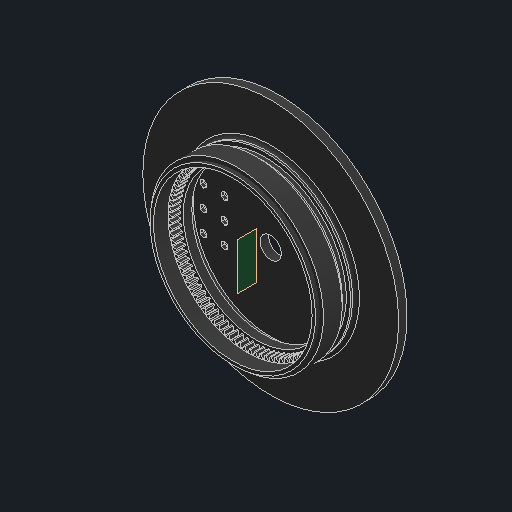
# Autodesk Inventor part: 스퍼 기어1
Saved by Autodesk Inventor 2026.1 (Build 301233020, 233B)
## iProperties
CustomPartVersion: 1
Created: 2025-11-12
Part Number: 스퍼 기어1
Material: 고무, 검은색
Document SubType Name: Modeling
Designer: jaewook
Categories: <?xml version="1.0" encoding="UTF-16"?> <MemberInstance><Categories><FamilyTemplate><FamilyTemplateParameter ValueType="xs:double" Id="1" ObjectReferenceKey="da_z" ObjectType="kUserParameterObject"/><FamilyTemplateParameter ValueType="xs:double" Id="2" ObjectReferenceKey="da_b" ObjectType="kUserParameterObject"/><FamilyTemplateParameter ValueType="xs:double" Id="3" ObjectReferenceKey="da_beta" ObjectType="kUserParameterObject"/><FamilyTemplateParameter ValueType="xs:double" Id="4" ObjectReferenceKey="da_da" ObjectType="kUserParameterObject"/><FamilyTemplateParameter ValueType="xs:double" Id="5" ObjectReferenceKey="da_aw" ObjectType="kUserParameterObject"/><FamilyTemplateParameter ValueType="xs:string" Id="6" ObjectReferenceKey="EAIAABAAAACIAQAAAAAAAIAAAAAAAAAA" ObjectType="83910656" SubObjectId="SurfaceGeometry"/></FamilyTemplate><ParamToTemplateMap><ParamToTemplate CategoryParameter="//CategoryParameter[@InternalName='046C89C9-8512-4d59-83FE-43B91F4F132A']" TemplateParameter="1"/><ParamToTemplate CategoryParameter="//CategoryParameter[@InternalName='2552DF32-E462-4b46-AEBF-C6C7768E72AC']" TemplateParameter="2"/><ParamToTemplate CategoryParameter="//CategoryParameter[@InternalName='C9EE641D-15FC-4fae-A226-E94C4372FDD7']" TemplateParameter="3"/><ParamToTemplate><ParamToTemplate CategoryParameter="//CategoryParameter[@InternalName='00B6519A-459B-49c7-AD84-2E56D39A5744']" ConstantValue="0.000000"/></ParamToTemplate><ParamToTemplate><ParamToTemplate CategoryParameter="//CategoryParameter[@InternalName='04B31F0E-C7A6-4894-AA32-9629BEFACF47']" ConstantValue="0.950000"/></ParamToTemplate><ParamToTemplate><ParamToTemplate CategoryParameter="//CategoryParameter[@InternalName='43CBEC2E-7847-49e7-A936-2F7889FCB2D9']" ConstantValue="0.250000"/></ParamToTemplate><ParamToTemplate><ParamToTemplate CategoryParameter="//CategoryParameter[@InternalName='B1EFC894-105D-4ebd-86BF-FA20ED196853']" ConstantValue="0.379900"/></ParamToTemplate><ParamToTemplate><ParamToTemplate CategoryParameter="//CategoryParameter[@InternalName='51175063-3D10-4879-93E8-6246FE8B403D']" ConstantValue="2060000000.000000"/></ParamToTemplate><ParamToTemplate><ParamToTemplate CategoryParameter="//CategoryParameter[@InternalName='A3A52E27-4454-46a9-B0BD-C932399B70AF']" ConstantValue="0.300000"/></ParamToTemplate><ParamToTemplate><ParamToTemplate CategoryParameter="//CategoryParameter[@InternalName='91B76062-C214-41d9-B1B9-14D2AB99603D']" ConstantValue="0.200000"/></ParamToTemplate><ParamToTemplate><ParamToTemplate CategoryParameter="//CategoryParameter[@InternalName='374E806E-8B8A-4dda-A9AA-1039D6500AD2']" ConstantValue="5.000000"/></ParamToTemplate><ParamToTemplate><ParamToTemplate CategoryParameter="//CategoryParameter[@InternalName='2D373A89-B862-43d6-8D0B-0CBF12AB9F6C']" ConstantValue="0.349066"/></ParamToTemplate><ParamToTemplate CategoryParameter="//CategoryParameter[@InternalName='37777632-D6A2-4fac-9D53-DB8ACD95C989']" TemplateParameter="4"/><ParamToTemplate CategoryParameter="//CategoryParameter[@InternalName='FD1017F1-B727-4f7e-9707-0F86F1FF9423']" TemplateParameter="5"/><ParamToTemplate><ParamToTemplate CategoryParameter="//CategoryParameter[@InternalName='9E1B4470-B2D3-4ff1-B813-535BB4CDF51A']" ConstantValue="3520000.000000"/></ParamToTemplate><ParamToTemplate><ParamToTemplate CategoryParameter="//CategoryParameter[@InternalName='F8452263-BFF6-458c-9FB1-07C4B99E95CD']" ConstantValue="11400000.000000"/></ParamToTemplate><ParamToTemplate><ParamToTemplate CategoryParameter="//CategoryParameter[@InternalName='3E3BB259-FD49-497f-8171-6EBC954A3479']" ConstantValue="2.000000"/></ParamToTemplate><ParamToTemplate CategoryParameter="//CategoryParameter[@InternalName='27C3BAF2-7550-4e4b-AE2C-0DB134B7D9B7']" TemplateParameter="6"/></ParamToTemplateMap><Category DisplayName="Gear" InternalName="DC85795E-93AB-48d5-8EEE-5A27447B64BD" Mnemonic="Gear"><CategoryParameter DisplayName="z" InternalName="046C89C9-8512-4d59-83FE-43B91F4F132A" Mnemonic="z"/><CategoryParameter DisplayName="b" InternalName="2552DF32-E462-4b46-AEBF-C6C7768E72AC" Mnemonic="b"/><CategoryParameter DisplayName="||b|" InternalName="C9EE641D-15FC-4fae-A226-E94C4372FDD7" Mnemonic="beta"/><CategoryParameter DisplayName="x" InternalName="00B6519A-459B-49c7-AD84-2E56D39A5744" Mnemonic="x"/><CategoryParameter DisplayName="a*" InternalName="04B31F0E-C7A6-4894-AA32-9629BEFACF47" Mnemonic="a"/><CategoryParameter DisplayName="c*" InternalName="43CBEC2E-7847-49e7-A936-2F7889FCB2D9" Mnemonic="c"/><CategoryParameter DisplayName="r|.f|*" InternalName="B1EFC894-105D-4ebd-86BF-FA20ED196853" Mnemonic="rf"/><CategoryParameter DisplayName="E" InternalName="51175063-3D10-4879-93E8-6246FE8B403D" Mnemonic="E"/><CategoryParameter DisplayName="||m|" InternalName="A3A52E27-4454-46a9-B0BD-C932399B70AF" Mnemonic="mi"/><Category DisplayName="SpurGear" InternalName="26C5A22E-A91E-4dfd-A3B3-23CCAFAE1764" Mnemonic="SpurGear"><CategoryParameter DisplayName="m" InternalName="91B76062-C214-41d9-B1B9-14D2AB99603D" Mnemonic="m"/><CategoryParameter DisplayName="P" InternalName="374E806E-8B8A-4dda-A9AA-1039D6500AD2" Mnemonic="PP"/><CategoryParameter DisplayName="||a|" InternalName="2D373A89-B862-43d6-8D0B-0CBF12AB9F6C" Mnemonic="alpha"/><CategoryParameter DisplayName="d|.a|" InternalName="37777632-D6A2-4fac-9D53-DB8ACD95C989" Mnemonic="da"/><CategoryParameter DisplayName="a|.w|" InternalName="FD1017F1-B727-4f7e-9707-0F86F1FF9423" Mnemonic="aw"/><CategoryParameter DisplayName="||s||.Flim|" InternalName="9E1B4470-B2D3-4ff1-B813-535BB4CDF51A" Mnemonic="sFlim"/><CategoryParameter DisplayName="||s||.Hlim|" InternalName="F8452263-BFF6-458c-9FB1-07C4B99E95CD" Mnemonic="sHlim"/><CategoryParameter DisplayName="유형" InternalName="3E3BB259-FD49-497f-8171-6EBC954A3479" Mnemonic="type"/><Category DisplayName="InternalSpurGear" InternalName="7CF704F6-14A9-42f8-93CE-E71DF57C2B55" Mnemonic="InternalSpurGear"><CategoryParameter DisplayName="PitchDiameter" InternalName="27C3BAF2-7550-4e4b-AE2C-0DB134B7D9B7" Mnemonic="IDS_PITCHDIAM"/></Category></Category></Category></Categories></MemberInstance>
Density: 0.93 g/cm^3
Appearance: 고무 - 검은색
d16: 70.000 mm
d17: 0.000 mm
d45: 0.000 mm
d47: 70.000 mm
d50: 0.000 mm
d51: 0.000 mm
d52: 70.000 mm
Author: jaewook
Autodesk Inventor part; units mm, degrees
sketch "Sketch1" plane through (0, 0, 0) normal (0, 0, 1) x (1, 0, 0)
  circle A0 centre (0, 0) radius 97.02
  dimension "d0" = 194.04
  constraints: 1 centre point
  measures "d0" diameter of A0
extrude "Extrusion1" add sketch "Sketch1" along normal blind 10
ref_plane "Work Plane2" through (0, 0, 5) normal (0, 0, 1) x (1, 0, 0)
sketch "Sketch2" plane through (0, 0, 0) normal (0, 0, -1) x (-1, 0, 0)
  circle A0 centre (0, 0) radius 97.02 projected
  circle A1 centre (0, 0) radius 90
  dimension "d3" = 180
  constraints: 1 centre point, 1 coincident
  measures "d3" diameter of A1
surface extrude "피치 지름" sketch "Sketch2" against normal through all shown no curves A1
ref_plane "Work Plane8" through (0, 0, 0) normal (0.9993908, 0.0348995, 0) x (0, 0, 1)
ref_plane "Work Plane9" through (0, 0, 0) normal (1, 0, 0) x (0, 1, 0)
spur gear teeth "스퍼 기어" teeth 90 pitch diameter 180 tip diameter 176.2 root diameter 184.8 face width 10 start plane through (0, 0, 0) normal (0, 0, -1) x (-1, 0, 0)
sketch "스케치14" plane through (0, 0, 10) normal (0, 0, 1) x (1, 0, 0)
  circle A0 centre (0, 0) radius 97.02 projected
  circle A1 centre (0, 0) radius 93.02
  dimension "d81" = 4
  constraints: 1 centre point, 1 coincident
  measures "d81" radial gap between concentric circles of A1 A0
extrude "돌출9" add sketch "스케치14" along normal blind 17
sketch "스케치15" plane through (0, 0, 0) normal (0, 0, -1) x (-1, 0, 0)
  circle A0 centre (0, 0) radius 97.02 projected
  circle A1 centre (0, 0) radius 92.4
  circle A2 centre (0, 0) radius 95.02
  circle A3 centre (0, 0) radius 85
  dimension "d84" = 184.8
  dimension "d85" = 190.04
  dimension "d86" = 170
  constraints: 3 centre point, 3 coincident
  measures "d84" diameter of A1
  measures "d85" diameter of A2
  measures "d86" diameter of A3
extrude "돌출10" add sketch "스케치15" along normal blind 10 contours A1 | A2
sketch "스케치16" plane through (0, 0, -10) normal (0, 0, -1) x (-1, 0, 0)
  circle A0 centre (0, 0) radius 95.02 projected
  circle A1 centre (0, 0) radius 85 projected
  circle A2 centre (0, 0) radius 90.78
  dimension "d89" = 4.24
  constraints: 1 centre point, 1 coincident
  measures "d89" radial gap between concentric circles of A2 A0
extrude "돌출11" add sketch "스케치16" along normal blind 1 contours A0
sketch "스케치17" plane through (0, 0, -11) normal (0, 0, -1) x (-1, 0, 0)
  circle A0 centre (0, 0) radius 90.78 projected
  circle A1 centre (0, 0) radius 85 projected
  circle A2 centre (0, 0) radius 100.02
  circle A3 centre (0, 0) radius 95.02 projected
  dimension "d150" = 5
  constraints: 1 centre point, 1 coincident
  measures "d150" radial gap between concentric circles of A2 A3
extrude "돌출12" add sketch "스케치17" along normal blind 6.5 contours A2 | A3
sketch "스케치18" plane through (0, 0, -17.5) normal (0, 0, -1) x (-1, 0, 0)
  circle A0 centre (0, 0) radius 90.78 projected
  circle A1 centre (0, 0) radius 150
  circle A2 centre (0, 0) radius 12.5
  dimension "d94" = 300
  dimension "d95" = 25
  constraints: 2 centre point, 2 coincident
  measures "d94" diameter of A1
  measures "d95" diameter of A2
extrude "돌출13" add sketch "스케치18" along normal blind 10 contours A0 | A1
fillet "모깎기2" radius 4 1 edges at (100.02, 0, -17.5)
sketch "스케치4" plane through (0, 0, 0) normal (0, 0, -1) x (-1, 0, 0)
  arc A0 (-13.6576, -91.3851) -> (-12.0606, -91.6095) centre (0, 0) ccw projected
  arc A1 (-19.999, -90.2098) -> (-18.4216, -90.545) centre (0, 0) ccw projected
  arc A2 (-26.243, -88.5949) -> (-24.6928, -89.0395) centre (0, 0) ccw projected
  arc A3 (-32.3592, -86.5485) -> (-30.8438, -87.1001) centre (0, 0) ccw projected
  arc A4 (-38.3177, -84.0804) -> (-36.8444, -84.7364) centre (0, 0) ccw projected
  arc A5 (-44.0895, -81.2027) -> (-42.6656, -81.9598) centre (0, 0) ccw projected
  arc A6 (-49.6465, -77.9294) -> (-48.2789, -78.784) centre (0, 0) ccw projected
  arc A7 (-54.9616, -74.2764) -> (-53.657, -75.2243) centre (0, 0) ccw projected
  arc A8 (-60.009, -70.2615) -> (-58.7736, -71.2981) centre (0, 0) ccw projected
  arc A9 (-64.764, -65.9043) -> (-63.604, -67.0246) centre (0, 0) ccw projected
  arc A10 (-69.2035, -61.2261) -> (-68.1244, -62.4245) centre (0, 0) ccw projected
  arc A11 (-73.3058, -56.2496) -> (-72.313, -57.5204) centre (0, 0) ccw projected
  arc A12 (-77.051, -50.999) -> (-76.1493, -52.3359) centre (0, 0) ccw projected
  arc A13 (-80.4209, -45.4999) -> (-79.6145, -46.8965) centre (0, 0) ccw projected
  arc A14 (-83.3989, -39.7792) -> (-82.6919, -41.2287) centre (0, 0) ccw projected
  arc A15 (-85.9706, -33.8647) -> (-85.3665, -35.3599) centre (0, 0) ccw projected
  arc A16 (-88.1234, -27.7852) -> (-87.6251, -29.319) centre (0, 0) ccw projected
  arc A17 (-89.847, -21.5704) -> (-89.4568, -23.1351) centre (0, 0) ccw projected
  arc A18 (-91.1328, -15.2504) -> (-90.8528, -16.8386) centre (0, 0) ccw projected
  arc A19 (-91.9746, -8.8561) -> (-91.806, -10.46) centre (0, 0) ccw projected
  arc A20 (-92.3683, -2.4188) -> (-92.3121, -4.0304) centre (0, 0) ccw projected
  arc A21 (-92.3121, 4.0304) -> (-92.3683, 2.4188) centre (0, 0) ccw projected
  arc A22 (-91.806, 10.46) -> (-91.9746, 8.8561) centre (0, 0) ccw projected
  arc A23 (-90.8528, 16.8386) -> (-91.1328, 15.2504) centre (0, 0) ccw projected
  arc A24 (-89.4568, 23.1351) -> (-89.847, 21.5704) centre (0, 0) ccw projected
  arc A25 (-87.6251, 29.319) -> (-88.1234, 27.7852) centre (0, 0) ccw projected
  arc A26 (-85.3665, 35.3599) -> (-85.9706, 33.8647) centre (0, 0) ccw projected
  arc A27 (-82.6919, 41.2287) -> (-83.3989, 39.7792) centre (0, 0) ccw projected
  arc A28 (-79.6145, 46.8965) -> (-80.4209, 45.4999) centre (0, 0) ccw projected
  arc A29 (-76.1493, 52.3359) -> (-77.051, 50.999) centre (0, 0) ccw projected
  arc A30 (-72.313, 57.5204) -> (-73.3058, 56.2496) centre (0, 0) ccw projected
  arc A31 (-68.1244, 62.4245) -> (-69.2035, 61.2261) centre (0, 0) ccw projected
  arc A32 (-63.604, 67.0246) -> (-64.764, 65.9043) centre (0, 0) ccw projected
  arc A33 (-58.7736, 71.2981) -> (-60.009, 70.2615) centre (0, 0) ccw projected
  arc A34 (-53.657, 75.2243) -> (-54.9616, 74.2764) centre (0, 0) ccw projected
  arc A35 (-48.2789, 78.784) -> (-49.6465, 77.9294) centre (0, 0) ccw projected
  arc A36 (-42.6656, 81.9598) -> (-44.0895, 81.2027) centre (0, 0) ccw projected
  arc A37 (-36.8444, 84.7364) -> (-38.3177, 84.0804) centre (0, 0) ccw projected
  arc A38 (-30.8438, 87.1001) -> (-32.3592, 86.5485) centre (0, 0) ccw projected
  arc A39 (-24.6928, 89.0395) -> (-26.243, 88.5949) centre (0, 0) ccw projected
  arc A40 (-18.4216, 90.545) -> (-19.999, 90.2098) centre (0, 0) ccw projected
  arc A41 (-12.0606, 91.6095) -> (-13.6576, 91.3851) centre (0, 0) ccw projected
  arc A42 (-5.6409, 92.2277) -> (-7.2496, 92.1152) centre (0, 0) ccw projected
  arc A43 (0.8063, 92.3965) -> (-0.8063, 92.3965) centre (0, 0) ccw projected
  arc A44 (7.2496, 92.1152) -> (5.6409, 92.2277) centre (0, 0) ccw projected
  arc A45 (13.6576, 91.3851) -> (12.0606, 91.6095) centre (0, 0) ccw projected
  arc A46 (19.999, 90.2098) -> (18.4216, 90.545) centre (0, 0) ccw projected
  arc A47 (26.243, 88.5949) -> (24.6928, 89.0395) centre (0, 0) ccw projected
  arc A48 (32.3592, 86.5485) -> (30.8438, 87.1001) centre (0, 0) ccw projected
  arc A49 (38.3177, 84.0804) -> (36.8444, 84.7364) centre (0, 0) ccw projected
  arc A50 (44.0895, 81.2027) -> (42.6656, 81.9598) centre (0, 0) ccw projected
  arc A51 (49.6465, 77.9294) -> (48.2789, 78.784) centre (0, 0) ccw projected
  arc A52 (54.9616, 74.2764) -> (53.657, 75.2243) centre (0, 0) ccw projected
  arc A53 (60.009, 70.2615) -> (58.7736, 71.2981) centre (0, 0) ccw projected
  arc A54 (64.764, 65.9043) -> (63.604, 67.0246) centre (0, 0) ccw projected
  arc A55 (69.2035, 61.2261) -> (68.1244, 62.4245) centre (0, 0) ccw projected
  arc A56 (73.3058, 56.2496) -> (72.313, 57.5204) centre (0, 0) ccw projected
  arc A57 (77.051, 50.999) -> (76.1493, 52.3359) centre (0, 0) ccw projected
  arc A58 (80.4209, 45.4999) -> (79.6145, 46.8965) centre (0, 0) ccw projected
  arc A59 (83.3989, 39.7792) -> (82.6919, 41.2287) centre (0, 0) ccw projected
  arc A60 (85.9706, 33.8647) -> (85.3665, 35.3599) centre (0, 0) ccw projected
  arc A61 (88.1234, 27.7852) -> (87.6251, 29.319) centre (0, 0) ccw projected
  arc A62 (89.847, 21.5704) -> (89.4568, 23.1351) centre (0, 0) ccw projected
  arc A63 (91.1328, 15.2504) -> (90.8528, 16.8386) centre (0, 0) ccw projected
  arc A64 (91.9746, 8.8561) -> (91.806, 10.46) centre (0, 0) ccw projected
  arc A65 (92.3683, 2.4188) -> (92.3121, 4.0304) centre (0, 0) ccw projected
  arc A66 (92.3121, -4.0304) -> (92.3683, -2.4188) centre (0, 0) ccw projected
  arc A67 (91.806, -10.46) -> (91.9746, -8.8561) centre (0, 0) ccw projected
  arc A68 (90.8528, -16.8386) -> (91.1328, -15.2504) centre (0, 0) ccw projected
  arc A69 (89.4568, -23.1351) -> (89.847, -21.5704) centre (0, 0) ccw projected
  arc A70 (87.6251, -29.319) -> (88.1234, -27.7852) centre (0, 0) ccw projected
  arc A71 (85.3665, -35.3599) -> (85.9706, -33.8647) centre (0, 0) ccw projected
  arc A72 (82.6919, -41.2287) -> (83.3989, -39.7792) centre (0, 0) ccw projected
  arc A73 (79.6145, -46.8965) -> (80.4209, -45.4999) centre (0, 0) ccw projected
  arc A74 (76.1493, -52.3359) -> (77.051, -50.999) centre (0, 0) ccw projected
  arc A75 (72.313, -57.5204) -> (73.3058, -56.2496) centre (0, 0) ccw projected
  arc A76 (68.1244, -62.4245) -> (69.2035, -61.2261) centre (0, 0) ccw projected
  arc A77 (63.604, -67.0246) -> (64.764, -65.9043) centre (0, 0) ccw projected
  arc A78 (58.7736, -71.2981) -> (60.009, -70.2615) centre (0, 0) ccw projected
  arc A79 (53.657, -75.2243) -> (54.9616, -74.2764) centre (0, 0) ccw projected
  arc A80 (48.2789, -78.784) -> (49.6465, -77.9294) centre (0, 0) ccw projected
  arc A81 (42.6656, -81.9598) -> (44.0895, -81.2027) centre (0, 0) ccw projected
  arc A82 (36.8444, -84.7364) -> (38.3177, -84.0804) centre (0, 0) ccw projected
  arc A83 (30.8438, -87.1001) -> (32.3592, -86.5485) centre (0, 0) ccw projected
  arc A84 (24.6928, -89.0395) -> (26.243, -88.5949) centre (0, 0) ccw projected
  arc A85 (18.4216, -90.545) -> (19.999, -90.2098) centre (0, 0) ccw projected
  arc A86 (12.0606, -91.6095) -> (13.6576, -91.3851) centre (0, 0) ccw projected
  arc A87 (5.6409, -92.2277) -> (7.2496, -92.1152) centre (0, 0) ccw projected
  arc A88 (-0.8063, -92.3965) -> (0.8063, -92.3965) centre (0, 0) ccw projected
  arc A89 (-7.2496, -92.1152) -> (-5.6409, -92.2277) centre (0, 0) ccw projected
  circle A90 centre (0, 0) radius 97.02 projected
  circle A91 centre (0, 0) radius 92.4
  point P0 (-92.3683, 2.4188)
  point P1 (-92.3121, 4.0304)
  point P2 (-91.9746, 8.8561)
  point P3 (-91.1328, 15.2504)
  point P4 (-89.847, 21.5704)
  point P5 (-88.1234, 27.7852)
  point P6 (-83.3989, 39.7792)
  point P7 (-80.4209, 45.4999)
  point P8 (-79.6145, 46.8965)
  point P9 (-76.1493, 52.3359)
  point P10 (-72.313, 57.5204)
  point P11 (-60.009, 70.2615)
  point P12 (-58.7736, 71.2981)
  point P13 (-54.9616, 74.2764)
  point P14 (-53.657, 75.2243)
  point P15 (-44.0895, 81.2027)
  point P16 (-38.3177, 84.0804)
  point P17 (-32.3592, 86.5485)
  point P18 (-26.243, 88.5949)
  point P19 (-24.6928, 89.0395)
  point P20 (-19.999, 90.2098)
  point P21 (-18.4216, 90.545)
  point P22 (-13.6576, 91.3851)
  point P23 (-12.0606, 91.6095)
  point P24 (-7.2496, 92.1152)
  point P25 (-0.8063, 92.3965)
  point P26 (0.8063, 92.3965)
  point P27 (5.6409, 92.2277)
  point P28 (7.2496, 92.1152)
  point P29 (12.0606, 91.6095)
  point P30 (18.4216, 90.545)
  point P31 (24.6928, 89.0395)
  point P32 (30.8438, 87.1001)
  point P33 (36.8444, 84.7364)
  point P34 (38.3177, 84.0804)
  point P35 (42.6656, 81.9598)
  point P36 (48.2789, 78.784)
  point P37 (49.6465, 77.9294)
  point P38 (54.9616, 74.2764)
  point P39 (58.7736, 71.2981)
  point P40 (63.604, 67.0246)
  point P41 (68.1244, 62.4245)
  point P42 (72.313, 57.5204)
  point P43 (73.3058, 56.2496)
  point P44 (79.6145, 46.8965)
  point P45 (80.4209, 45.4999)
  point P46 (85.3665, 35.3599)
  point P47 (87.6251, 29.319)
  point P48 (89.4568, 23.1351)
  point P49 (89.847, 21.5704)
  point P50 (90.8528, 16.8386)
  point P51 (91.1328, 15.2504)
  point P52 (91.806, 10.46)
  point P53 (91.9746, 8.8561)
  point P54 (92.3683, -2.4188)
  point P55 (92.3121, -4.0304)
  point P56 (91.9746, -8.8561)
  point P57 (91.1328, -15.2504)
  point P58 (89.847, -21.5704)
  point P59 (88.1234, -27.7852)
  point P60 (85.9706, -33.8647)
  point P61 (72.313, -57.5204)
  point P62 (60.009, -70.2615)
  point P63 (58.7736, -71.2981)
  point P64 (54.9616, -74.2764)
  point P65 (53.657, -75.2243)
  point P66 (49.6465, -77.9294)
  point P67 (44.0895, -81.2027)
  point P68 (38.3177, -84.0804)
  point P69 (32.3592, -86.5485)
  point P70 (26.243, -88.5949)
  point P71 (19.999, -90.2098)
  point P72 (18.4216, -90.545)
  point P73 (13.6576, -91.3851)
  point P74 (12.0606, -91.6095)
  point P75 (7.2496, -92.1152)
  point P76 (0.8063, -92.3965)
  point P77 (-0.8063, -92.3965)
  point P78 (-7.2496, -92.1152)
  point P79 (-12.0606, -91.6095)
  point P80 (-18.4216, -90.545)
  point P81 (-24.6928, -89.0395)
  point P82 (-26.243, -88.5949)
  point P83 (-30.8438, -87.1001)
  point P84 (-32.3592, -86.5485)
  point P85 (-36.8444, -84.7364)
  point P86 (-38.3177, -84.0804)
  point P87 (-48.2789, -78.784)
  point P88 (-53.657, -75.2243)
  point P89 (-58.7736, -71.2981)
  point P90 (-63.604, -67.0246)
  point P91 (-64.764, -65.9043)
  point P92 (-69.2035, -61.2261)
  point P93 (-72.313, -57.5204)
  point P94 (-73.3058, -56.2496)
  point P95 (-76.1493, -52.3359)
  point P96 (-77.051, -50.999)
  point P97 (-82.6919, -41.2287)
  point P98 (-83.3989, -39.7792)
  point P99 (-85.3665, -35.3599)
  point P100 (-87.6251, -29.319)
  point P101 (-90.8528, -16.8386)
  point P102 (-91.806, -10.46)
  point P103 (-92.3121, -4.0304)
  constraints: 1 coincident, 1 other
sketch "스케치6" plane through (0, 0, -10) normal (0, 0, -1) x (-1, 0, 0)
  arc A0 (51.6266, -76.6319) -> (92.1785, -6.394) centre (0, 0) ccw projected
  circle A1 centre (0, 0) radius 101.64 projected
  arc A2 (92.1785, 6.394) -> (51.6266, 76.6319) centre (0, 0) ccw projected
  circle A3 centre (0, 0) radius 97.02
  dimension "d69" = 4.62
  constraints: 1 centre point, 1 coincident
  measures "d69" radial gap between concentric circles of A0 A3
sketch "스케치7" plane through (0, 0, -10) normal (0, 0, -1) x (-1, 0, 0)
  circle A0 centre (0, 0) radius 97.02 projected
  arc A1 (51.6266, -76.6319) -> (92.1785, -6.394) centre (0, 0) ccw projected
  arc A2 (-40.5519, -83.0259) -> (40.5519, -83.0259) centre (0, 0) ccw projected
  arc A3 (-92.1785, -6.394) -> (-51.6266, -76.6319) centre (0, 0) ccw projected
  arc A4 (-51.6266, 76.6319) -> (-92.1785, 6.394) centre (0, 0) ccw projected
  arc A5 (40.5519, 83.0259) -> (-40.5519, 83.0259) centre (0, 0) ccw projected
  arc A6 (92.1785, 6.394) -> (51.6266, 76.6319) centre (0, 0) ccw projected
  circle A7 centre (0, 0) radius 97.02
  circle A8 centre (0, 0) radius 92.4
  point P0 (-92.1785, -6.394)
  point P1 (-92.1785, 6.394)
  point P2 (-51.6266, 76.6319)
  point P3 (-40.5519, 83.0259)
  point P4 (40.5519, 83.0259)
  point P5 (92.1785, 6.394)
  point P6 (40.5519, -83.0259)
  point P7 (-40.5519, -83.0259)
  point P8 (-51.6266, -76.6319)
  constraints: 2 centre point, 2 coincident, 2 concentric
sketch "스케치8" plane through (0, 0, -14) normal (0, 0, -1) x (-1, 0, 0)
  circle A0 centre (0, 0) radius 97.02 projected
  circle A1 centre (0, 0) radius 92.4 projected
  circle A2 centre (0, 0) radius 102.45
  constraints: 1 centre point, 1 coincident
sketch "스케치9" plane through (0, 0, -14) normal (0, 0, 1) x (1, 0, 0)
  circle A0 centre (0, 0) radius 102.45 projected
  circle A1 centre (0, 0) radius 97.02 projected
sketch "스케치10" plane through (0, 0, -18) normal (0, 0, -1) x (-1, 0, 0)
  circle A0 centre (0, 0) radius 102.45 projected
  circle A1 centre (0, 0) radius 92.4 projected
  circle A2 centre (0, 0) radius 150
  dimension "d78" = 300
  constraints: 1 centre point, 1 coincident
  measures "d78" diameter of A2
mirror "미러1" about plane through (0, 0, 0) normal (1, 0, 0)
sketch "스케치25" plane through (0, 0, -27.5) normal (0, 0, -1) x (-1, 0, 0)
  circle A0 centre (0, 0) radius 150 projected
  circle A1 centre (0, 0) radius 12.5 projected
  line L0 (59, -80) -> (74, -80)
  line L1 (74, -80) -> (74, 80)
  line L2 (74, 80) -> (59, 80)
  line L3 (59, 80) -> (59, -80)
  line L4 (0, 0) -> (150, 0) construction
  line L5 (0, 0) -> (0, 150) construction
  line L6 (-59, -80) -> (-74, -80)
  line L7 (-74, -80) -> (-74, 80)
  line L8 (-74, 80) -> (-59, 80)
  line L9 (-59, 80) -> (-59, -80)
  line L10 (74, -39.75) -> (127.216, -39.75)
  line L11 (127.216, -39.75) -> (127.216, -30.25)
  line L12 (127.216, -30.25) -> (74, -30.25)
  line L13 (74, -30.25) -> (74, -39.75)
  line L14 (74, 39.75) -> (127.216, 39.75)
  line L15 (127.216, 39.75) -> (127.216, 30.25)
  line L16 (127.216, 30.25) -> (74, 30.25)
  line L17 (74, 30.25) -> (74, 39.75)
  line L18 (-74, -39.75) -> (-127.216, -39.75)
  line L19 (-127.216, -39.75) -> (-127.216, -30.25)
  line L20 (-127.216, -30.25) -> (-74, -30.25)
  line L21 (-74, -30.25) -> (-74, -39.75)
  line L22 (-74, 30.25) -> (-74, 39.75)
  line L23 (-74, 39.75) -> (-127.216, 39.75)
  line L24 (-127.216, 39.75) -> (-127.216, 30.25)
  line L25 (-127.216, 30.25) -> (-74, 30.25)
  dimension "d139" = 59
  dimension "d140" = 15
  dimension "d141" = 160
  dimension "d163" = 9.5
  dimension "d164" = 40.25
  dimension "d165" = 53.216
  constraints: 52 end point, 16 symmetric about line, 4 parallel, 2 horizontal, 2 perpendicular, 2 point on circle, 1 point on line, 1 vertical, 1 other
  measures "d139" distance from line of L3 A0.centre
  measures "d140" distance of L1.end L2.end
  measures "d141" distance of L0.end L1.end
  measures "d163" distance of L11.end L10.end
  measures "d164" distance between parallel lines of L10 L0
  measures "d165" distance between parallel lines of L11 L1
extrude "돌출19" cut sketch "스케치25" against normal blind 5 contours L3 L2 L1 L0 | L1 L12 L11 L10 | L14 L15 L16 L1 | L6 L7 L8 L9 | L18 L19 L20 L7 | L7 L25 L24 L23
sketch "스케치29" plane through (0, 0, 0) normal (1, 0, 0) x (0, 1, 0)
  line L0 (-100.02, -11) -> (100.02, -11) projected
  line L1 (101.32, 0) -> (95.02, -6.3)
  line L2 (-97.02, 0) -> (97.02, 0) projected
  line L3 (95.02, 0) -> (95.02, -11) projected
  line L4 (95.02, 0) -> (95.02, -11) projected
  line L5 (0, -11) -> (0, 0)
  line L6 (101.32, 0) -> (97.02, 0)
  point P0 (97.3, -4.02)
  point P1 (97.3, -4.02)
  dimension "d153" = 6.98
  dimension "d154" = 45
  dimension "d155" = 194.6
  constraints: 6 end point, 2 point on line, 1 coincident, 1 horizontal, 1 midpoint, 1 perpendicular
  measures "d153" distance from line of point (97.3, -4.02) L0
  measures "d154" angle of L2 L1
  measures "d155" diameter of point (97.3, -4.02) L5
revolve "회전2" add sketch "스케치29" angle 360 about axis through (0, 0, -11) along (0, 0, 1) separate body contours L3 L2 L6 L1
sketch "스케치30" plane through (0, 0, 0) normal (0, 0, 1) x (1, 0, 0)
  circle A0 centre (0, 0) radius 95.02 projected
  circle A1 centre (0, 0) radius 101.32 projected
extrude "돌출22" add sketch "스케치30" along normal blind 22 bodies 2
sketch "스케치31" plane through (0, 0, -27.5) normal (0, 0, -1) x (-1, 0, 0)
  line L0 (74, -80) -> (59, -80) projected
  line L1 (59, 80) -> (74, 80) projected
  line L2 (74, -30.25) -> (127.216, -30.25) projected
  circle A0 centre (0, 0) radius 12.5 projected
  line L3 (74, -30.25) -> (84, -30.25)
  line L4 (84, -30.25) -> (84, -20.25)
  line L5 (84, -20.25) -> (74, -20.25)
  line L6 (74, -20.25) -> (74, -30.25)
  line L7 (74, -30.25) -> (84, -20.25) construction
  line L8 (74, -20.25) -> (84, -30.25) construction
  line L9 (79, -20.9199) -> (82.75, -23.0849)
  line L10 (82.75, -23.0849) -> (82.75, -27.4151)
  line L11 (82.75, -27.4151) -> (79, -29.5801)
  line L12 (79, -29.5801) -> (75.25, -27.4151)
  line L13 (75.25, -27.4151) -> (75.25, -23.0849)
  line L14 (75.25, -23.0849) -> (79, -20.9199)
  line L15 (0, 0) -> (28.2657, 0) construction
  line L16 (0, 0) -> (0, 17.7241) construction
  line L17 (79, 20.9199) -> (82.75, 23.0849)
  line L18 (82.75, 23.0849) -> (82.75, 27.4151)
  line L19 (82.75, 27.4151) -> (79, 29.5801)
  line L20 (79, 29.5801) -> (75.25, 27.4151)
  line L21 (75.25, 27.4151) -> (75.25, 23.0849)
  line L22 (75.25, 23.0849) -> (79, 20.9199)
  line L23 (66.5, -80) -> (66.5, 80) construction
  line L24 (54, -20.9199) -> (50.25, -23.0849)
  line L25 (50.25, -23.0849) -> (50.25, -27.4151)
  line L26 (50.25, -27.4151) -> (54, -29.5801)
  line L27 (54, -29.5801) -> (57.75, -27.4151)
  line L28 (57.75, -27.4151) -> (57.75, -23.0849)
  line L29 (57.75, -23.0849) -> (54, -20.9199)
  line L30 (57.75, 27.4151) -> (57.75, 23.0849)
  line L31 (57.75, 23.0849) -> (54, 20.9199)
  line L32 (54, 29.5801) -> (57.75, 27.4151)
  line L33 (54, 20.9199) -> (50.25, 23.0849)
  line L34 (50.25, 23.0849) -> (50.25, 27.4151)
  line L35 (50.25, 27.4151) -> (54, 29.5801)
  line L36 (-79, -20.9199) -> (-82.75, -23.0849)
  line L37 (-82.75, -23.0849) -> (-82.75, -27.4151)
  line L38 (-82.75, -27.4151) -> (-79, -29.5801)
  line L39 (-79, -29.5801) -> (-75.25, -27.4151)
  line L40 (-75.25, -27.4151) -> (-75.25, -23.0849)
  line L41 (-75.25, -23.0849) -> (-79, -20.9199)
  line L42 (-75.25, 27.4151) -> (-75.25, 23.0849)
  line L43 (-75.25, 23.0849) -> (-79, 20.9199)
  line L44 (-79, 29.5801) -> (-75.25, 27.4151)
  line L45 (-79, 20.9199) -> (-82.75, 23.0849)
  line L46 (-82.75, 23.0849) -> (-82.75, 27.4151)
  line L47 (-82.75, 27.4151) -> (-79, 29.5801)
  line L48 (-54, -20.9199) -> (-50.25, -23.0849)
  line L49 (-57.75, -23.0849) -> (-54, -20.9199)
  line L50 (-50.25, -23.0849) -> (-50.25, -27.4151)
  line L51 (-57.75, -27.4151) -> (-57.75, -23.0849)
  line L52 (-50.25, -27.4151) -> (-54, -29.5801)
  line L53 (-54, -29.5801) -> (-57.75, -27.4151)
  line L54 (-57.75, 27.4151) -> (-57.75, 23.0849)
  line L55 (-57.75, 23.0849) -> (-54, 20.9199)
  line L56 (-54, 29.5801) -> (-57.75, 27.4151)
  line L57 (-54, 20.9199) -> (-50.25, 23.0849)
  line L58 (-50.25, 23.0849) -> (-50.25, 27.4151)
  line L59 (-50.25, 27.4151) -> (-54, 29.5801)
  line L60 (79, 25.25) -> (79, -25.25) construction
  line L61 (79, 4.3301) -> (82.75, 2.1651)
  line L62 (82.75, 2.1651) -> (82.75, -2.1651)
  line L63 (82.75, -2.1651) -> (79, -4.3301)
  line L64 (79, -4.3301) -> (75.25, -2.1651)
  line L65 (75.25, -2.1651) -> (75.25, 2.1651)
  line L66 (75.25, 2.1651) -> (79, 4.3301)
  line L67 (54, 4.3301) -> (50.25, 2.1651)
  line L68 (50.25, 2.1651) -> (50.25, -2.1651)
  line L69 (50.25, -2.1651) -> (54, -4.3301)
  line L70 (54, -4.3301) -> (57.75, -2.1651)
  line L71 (57.75, -2.1651) -> (57.75, 2.1651)
  line L72 (57.75, 2.1651) -> (54, 4.3301)
  line L73 (-79, 4.3301) -> (-82.75, 2.1651)
  line L74 (-82.75, 2.1651) -> (-82.75, -2.1651)
  line L75 (-82.75, -2.1651) -> (-79, -4.3301)
  line L76 (-79, -4.3301) -> (-75.25, -2.1651)
  line L77 (-75.25, -2.1651) -> (-75.25, 2.1651)
  line L78 (-75.25, 2.1651) -> (-79, 4.3301)
  line L79 (-57.75, -2.1651) -> (-57.75, 2.1651)
  line L80 (-50.25, 2.1651) -> (-50.25, -2.1651)
  line L81 (-57.75, 2.1651) -> (-54, 4.3301)
  line L82 (-54, 4.3301) -> (-50.25, 2.1651)
  line L83 (-54, -4.3301) -> (-57.75, -2.1651)
  line L84 (-50.25, -2.1651) -> (-54, -4.3301)
  circle A1 centre (-79, 25.25) radius 1.9
  circle A2 centre (-54, 25.25) radius 1.9
  circle A3 centre (-79, 0) radius 1.9
  circle A4 centre (-54, 0) radius 1.9
  circle A5 centre (-54, -25.25) radius 1.9
  circle A6 centre (-79, -25.25) radius 1.9
  circle A7 centre (54, 25.25) radius 1.9
  circle A8 centre (79, 25.25) radius 1.9
  circle A9 centre (54, 0) radius 1.9
  circle A10 centre (54, -25.25) radius 1.9
  circle A11 centre (79, -25.25) radius 1.9
  circle A12 centre (79, 0) radius 1.9
  point P0 (54, -25.25)
  point P1 (54, 25.25)
  point P2 (-79, -25.25)
  point P3 (-54, -25.25)
  point P4 (-54, 25.25)
  point P5 (54, 0)
  point P6 (-79, 0)
  point P7 (-54, 0)
  dimension "d166" = 10
  dimension "d167" = 10
  dimension "d168" = 7.5
  dimension "d169" = 7.5
  dimension "d172" = 3.8
  dimension "d173" = 3.8
  dimension "d174" = 3.8
  dimension "d175" = 3.8
  dimension "d176" = 3.8
  dimension "d177" = 3.8
  dimension "d178" = 3.8
  dimension "d179" = 3.8
  dimension "d180" = 3.8
  dimension "d181" = 3.8
  dimension "d182" = 3.8
  dimension "d183" = 3.8
  dimension "d56" = 238.049
  dimension "d57" = 255.5606
  dimension "d60" = 360
  dimension "d64" = 360
  constraints: 164 end point, 70 symmetric about line, 12 centre point, 4 midpoint, 3 coincident, 3 vertical, 2 horizontal, 2 parallel, 2 perpendicular, 2 point on line, 26 other
  measures "d166" distance of L5.end L4.end
  measures "d167" distance of L4.end L3.end
  measures "d168" distance between parallel lines of L10 L13
  measures "d169" distance between parallel lines of L62 L65
  measures "d172" diameter of A1
  measures "d173" diameter of A2
  measures "d174" diameter of A3
  measures "d175" diameter of A4
  measures "d176" diameter of A5
  measures "d177" diameter of A6
  measures "d178" diameter of A7
  measures "d179" diameter of A8
  measures "d180" diameter of A9
  measures "d181" diameter of A10
  measures "d182" diameter of A11
  measures "d183" diameter of A12
extrude "돌출23" cut sketch "스케치31" along normal blind 4 from surface at -10 contours L9 L10 L11 L12 L13 L14 | L22 L21 L20 L19 L18 L17 | L29 L28 L27 L26 L25 L24 | L30 L31 L33 L34 L35 L32 | L41 L40 L39 L38 L37 L36 | L42 L43 L45 L46 L47 L44 | L48 L50 L52 L53 L51 L49 | L56 L59 L58 L57 L55 L54 | L61 L62 L63 L64 L65 L66 | L72 L71 L70 L69 L68 L67 | L78 L77 L76 L75 L74 L73 | L79 L81 L82 L80 L84 L83 | A1 | A2 | A3 | A4 | A5 | A6 | A7 | A8 | A9 | A10 | A11 | A12 bodies 1
extrude "돌출24" cut sketch "스케치31" against normal through all contours A1 | A2 | A3 | A4 | A5 | A6 | A7 | A8 | A9 | A10 | A11 | A12 bodies 1
ref_plane "작업 평면12" through (0, 0, 0) normal (1, 0, 0) x (0, 1, 0)
equation "\"d1\" = da_b"
equation "\"d3\" = da_d"
equation "\"d16\" = da_aw"
equation "\"d47\" = da_aw"
equation "\"d52\" = da_aw"
equation "\"da_b\" = 10"
equation "\"da_d\" = 180"
equation "\"da_aw\" = 70"
body "Solid1"
body "Srf1"
